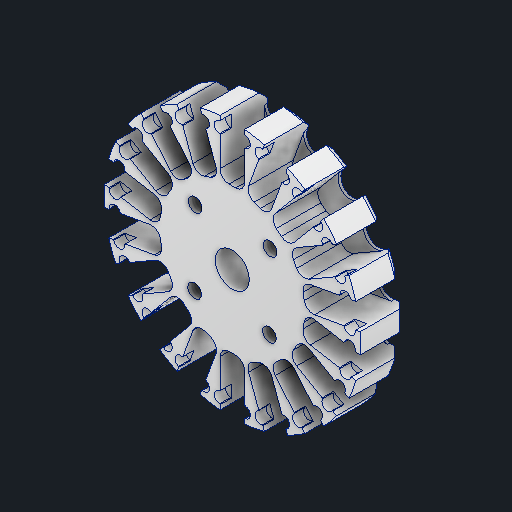
# Autodesk Inventor part: RadNeu
Saved by Autodesk Inventor 2025.2 (Build 292293000, 293)
## iProperties
Created: 2025-03-22
Part Number: RadNeu
Material: Generisch
Document SubType Name: Modeling
Designer: Faabs
Density: 1 g/cm^3
Appearance: Aluminium - flach
Author: Faabs
Autodesk Inventor part; units mm, degrees
ref_plane "YZ Plane" through (0, 0, 0) normal (1, 0, 0) x (0, 1, 0)
ref_plane "XZ Plane" through (0, 0, 0) normal (0, 1, 0) x (-1, 0, 0)
sketch "Skizze2" plane through (0, 0, 0) normal (0, -1, 0) x (1, 0, 0)
  circle A0 centre (0, 0) radius 13 construction
  circle A1 centre (0, 0) radius 23 projected
  line L0 (0, 0) -> (0, 23) construction
  line L1 (0, 23) -> (0, 13) construction
  line L2 (0, 13) -> (-0.6, 13)
  line L3 (-2.2, 14.6) -> (-2.2, 23)
  line L4 (-2.2, 23) -> (0, 23)
  line L5 (0, 23) -> (0, 13) construction
  line L6 (0, 13) -> (0.6, 13)
  line L7 (2.2, 14.6) -> (2.2, 23)
  line L8 (2.2, 23) -> (0, 23)
  arc A2 (-2.2, 14.6) -> (-0.6, 13) centre (-0.6, 14.6) ccw
  arc A3 (0.6, 13) -> (2.2, 14.6) centre (0.6, 14.6) ccw
  point P0 (2.2, 22.8945)
  point P1 (-2.2, 22.8945)
  dimension "d18" = 26
  dimension "d20" = 4.4
  dimension "d21" = 2.2
  dimension "d22" = 1.6
  dimension "d98" = 8.4
  constraints: 18 end point, 4 parallel, 4 point on circle, 4 tangent, 2 centre point, 2 perpendicular, 1 coincident, 1 collinear, 1 equal radius, 1 point on line, 1 vertical, 1 vertical alignment, 4 other
  measures "d20" distance between parallel lines of L3 L7
  measures "d21" distance between parallel lines of L0 L7
  measures "d22" radius of A2
  measures "d98" distance from line of L8 A3.centre
sketch "Skizze1" plane through (0, 0, 0) normal (0, 0, 1) x (1, 0, 0)
  line L0 (0, 0) -> (0, 8.5)
  line L1 (3.05, 0) -> (3.05, 8.5)
  line L2 (23, 0) -> (23, 8.5)
  line L3 (0, 0) -> (23, 0)
  line L4 (3.05, 8.5) -> (23, 8.5)
  dimension "d1" = 8.5
  dimension "d10" = 8.5
  dimension "d11" = 6.1
  dimension "d14" = 8.5
  dimension "d15" = 46
  constraints: 10 end point, 3 vertical, 2 horizontal
  measures "d1" distance of L0.start L0.end
  measures "d10" distance of L1.start L1.end
  measures "d11" diameter of L1 L0
  measures "d14" distance of L2.start L2.end
  measures "d15" diameter of L2 L0
revolve "Radkörper" add sketch "Skizze1" angle 360 about axis through (0, 0, 0) along (0, 1, 0)
extrude "Querrolle" cut sketch "Skizze2" against normal blind 8 contours L7 A3 L6 L2 A2 L3 A1 picked at (0, 17.4)
sketch "Skizze4" plane through (0, 0, 0) normal (0, -1, 0) x (1, 0, 0)
  line L0 (0.6, 13) -> (-0.6, 13) projected
  line L1 (0, 13) -> (0, 21) construction
  line L2 (-2.25, 22) -> (2.25, 22)
  line L3 (3.25, 21) -> (3.25, 21)
  line L4 (2.25, 20) -> (-2.25, 20)
  line L5 (-3.25, 21) -> (-3.25, 21)
  line L6 (-3.25, 22) -> (3.25, 20) construction
  line L7 (3.25, 22) -> (-3.25, 20) construction
  arc A0 (3.25, 21) -> (2.25, 22) centre (2.25, 21) ccw
  arc A1 (2.25, 20) -> (3.25, 21) centre (2.25, 21) ccw
  arc A2 (-3.25, 21) -> (-2.25, 20) centre (-2.25, 21) ccw
  arc A3 (-2.25, 22) -> (-3.25, 21) centre (-2.25, 21) ccw
  point P0 (0, 0)
  dimension "d25" = 8
  dimension "d26" = 6.5
  dimension "d27" = 2
  dimension "d28" = 1
  constraints: 14 end point, 8 point on circle, 8 point on line, 8 tangent, 4 centre point, 3 equal radius, 3 midpoint, 2 parallel, 1 horizontal, 1 perpendicular, 1 vertical
  measures "d25" distance of L1.start L1.end
  measures "d26" distance of L6.end L7.end
  measures "d27" distance of L7.start L6.end
  measures "d28" radius of A0
extrude "Achse" cut sketch "Skizze4" against normal blind 2
fillet "Rundung1" radius 0.1 4 edges at (-2.2, 1, 22) (2.2, 1, 22) (-2.2, 1, 20) (2.2, 1, 20)
pattern_circular "Runde Anordnung1" count 18 over 360 about axis through (0, -10, 0) along (0, 1, 0) of "Querrolle", "Achse", "Rundung1"
chamfer "Fasen1" distance 1.5 angle 45 1 edges at (-23, 8.5, 0)
sketch "Skizze6" plane through (0.6, 0, 14.6) normal (0, -1, 0) x (0.7071068, 0, -0.7071068)
  circle A0 centre (9.8995, -10.748) radius 9.5 construction
  line L0 (9.8995, -10.748) -> (0.7778, -1.4849) construction
  line L1 (0.4243, -1.8385) -> (1.1314, -1.1314) projected
  line L2 (9.8995, -10.748) -> (0.3998, -10.6749) construction
  point P0 (9.8264, -20.2477)
  point P1 (19.3992, -10.8211)
  point P2 (9.9726, -1.2483)
  dimension "d60" = 19
  dimension "d65" = 45
  dimension "d68" = 360
  constraints: 4 end point, 2 coincident, 1 midpoint, 8 other
  measures "d65" angle of L0 L2
hole "Bohrung1" at (-6.6656, 0, 6.769) at (6.769, 0, 6.6656) at (6.6656, 0, -6.769) at (-6.769, 0, -6.6656) direction (0, 1, 0) diameter 2.459 depth 6 tip angle 118 thread size "M3x0.5" class "6H" standard "ISO Metric profile"
sketch "Skizze12" plane through (0, 8, 0) normal (0, -1, 0) x (1, 0, 0)
  circle A0 centre (0, 0) radius 23
  line L0 (0, 23) -> (0, 20.5)
  arc A1 (-2.2, 20.5) -> (2.2, 20.5) centre (0, 20.5) ccw
  line L1 (-2.2, 14.6) -> (-2.2, 21.8897) projected
  line L2 (-2.2, 20.5) -> (-2.2, 22.8945)
  line L3 (2.2, 20.5) -> (2.2, 22.8945)
  arc A2 (-2.2955, 21.999) -> (-2.2955, 20.001) centre (-2.25, 21) ccw projected
  dimension "d85" = 46
  dimension "d86" = 2.5
  dimension "d100" = 2.2
  constraints: 6 end point, 5 point on circle, 2 centre point, 2 coincident, 2 point on line, 2 tangent, 1 parallel, 1 vertical
  measures "d85" diameter of A0
  measures "d86" distance of L0.start L0.end
  measures "d100" radius of A1
extrude "Durchbruch" cut sketch "Skizze12" against normal up to surface (0.5 mm away) contours L3 A1 L1 L2 A0 picked at (0, 21.3333)
pattern_circular "Runde Anordnung4" count 18 over 360 about axis through (0, -10, 0) along (0, 1, 0) of "Durchbruch", "Querrolle"
sketch "Skizze7" plane through (0.6, 0, 14.6) normal (0, -1, 0) x (0.7071068, 0, -0.7071068)
  circle A0 centre (0.3998, -10.6749) radius 1.2295 projected
  circle A1 centre (9.9726, -1.2483) radius 1.2295 projected
  circle A2 centre (19.3992, -10.8211) radius 1.2295 projected
  circle A3 centre (9.8264, -20.2477) radius 1.2295 projected
  point P0 (9.8995, -10.748)
  constraints: 4 coincident
hole "Durchgangsbohrung" [suppressed]
sketch "Skizze8" plane through (2.2, 8.5, -14.6) normal (0, 1, 0) x (1, 0, 0)
  line L0 (-2.2, -14.6) -> (-2.2, -17.65) construction
  circle A0 centre (-2.2, -14.6) radius 3.05 construction
  line L1 (-2.2, -14.6) -> (-4.3567, -16.7567) construction
  circle A1 centre (4.569, -21.2656) radius 1.55 projected
  line L2 (2.3236, -23.511) -> (1.5018, -20.4438)
  line L3 (1.5018, -20.4438) -> (3.7471, -18.1984)
  line L4 (3.7471, -18.1984) -> (6.8144, -19.0203)
  line L5 (6.8144, -19.0203) -> (7.6362, -22.0875)
  line L6 (7.6362, -22.0875) -> (5.3908, -24.3329)
  line L7 (5.3908, -24.3329) -> (2.3236, -23.511)
  line L8 (6.711, -10.0764) -> (3.6438, -10.8982)
  line L9 (3.6438, -10.8982) -> (1.3984, -8.6529)
  line L10 (1.3984, -8.6529) -> (2.2203, -5.5856)
  line L11 (2.2203, -5.5856) -> (5.2875, -4.7638)
  line L12 (5.2875, -4.7638) -> (7.5329, -7.0092)
  line L13 (7.5329, -7.0092) -> (6.711, -10.0764)
  line L14 (-6.7236, -5.689) -> (-5.9018, -8.7562)
  line L15 (-5.9018, -8.7562) -> (-8.1471, -11.0016)
  line L16 (-8.1471, -11.0016) -> (-11.2144, -10.1797)
  line L17 (-11.2144, -10.1797) -> (-12.0362, -7.1125)
  line L18 (-12.0362, -7.1125) -> (-9.7908, -4.8671)
  line L19 (-9.7908, -4.8671) -> (-6.7236, -5.689)
  line L20 (-11.111, -19.1236) -> (-8.0438, -18.3018)
  line L21 (-8.0438, -18.3018) -> (-5.7984, -20.5471)
  line L22 (-5.7984, -20.5471) -> (-6.6203, -23.6144)
  line L23 (-6.6203, -23.6144) -> (-9.6875, -24.4362)
  line L24 (-9.6875, -24.4362) -> (-11.9329, -22.1908)
  line L25 (-11.9329, -22.1908) -> (-11.111, -19.1236)
  point P0 (4.4656, -7.831)
  point P1 (-8.969, -7.9344)
  point P2 (-8.8656, -21.369)
  dimension "d77" = 45
  dimension "d78" = 5.5
  dimension "d81" = 360
  constraints: 52 end point, 2 point on circle, 1 coincident, 1 parallel, 1 vertical, 66 other
  measures "d77" angle of L0 L1
  measures "d78" distance between parallel lines of L6 L3
extrude "Muttern" [suppressed]
fillet "Rundung4" [suppressed]
fillet "Rundung5" [suppressed]
sketch "Skizze13" plane through (2.2, 0, 14.6) normal (0, -1, 0) x (1, 0, 0)
  circle A0 centre (-2.2, -14.6) radius 4.05
  arc A1 (-3.0292, -13.35) -> (-1.3708, -13.35) centre (-2.2, -14.6) ccw
  line L0 (-3.0292, -13.35) -> (-1.3708, -13.35)
  line L1 (-1.3268, -13.2) -> (-3.0732, -13.2)
  arc A2 (-3.0732, -13.2) -> (-1.3268, -13.2) centre (-2.2, -14.6) ccw
  dimension "d101" = 3
  dimension "d105" = 2.75
  dimension "d117" = 0.15
  constraints: 4 end point, 4 point on circle, 3 centre point, 2 coincident, 1 horizontal, 1 other
  measures "d101" diameter of A1
  measures "d117" distance between parallel lines of L0 L1
extrude "Extrusion5" [suppressed]
ref_plane "Arbeitsebene1" through (0, 0, 3) normal (0, 0, 1) x (1, 0, 0)
sketch "Skizze14" plane through (0, 0, 3) normal (0, 0, 1) x (1, 0, 0)
  line L0 (-2.2, 8.5) -> (2.2, 8.5) projected
  line L1 (0, 8.5) -> (0, 0)
  line L2 (2.5, 7.0566) -> (2.5, 4.1699)
  line L3 (2.5, 4.1699) -> (0, 2.7265)
  line L4 (0, 2.7265) -> (-2.5, 4.1699)
  line L5 (-2.5, 4.1699) -> (-2.5, 7.0566)
  line L6 (-2.5, 7.0566) -> (0, 8.5)
  line L7 (0, 8.5) -> (2.5, 7.0566)
  line L8 (2.5, 4.1699) -> (2.5, 8.5)
  line L9 (2.5, 8.5) -> (-2.5, 8.5)
  line L10 (-2.5, 8.5) -> (-2.5, 4.1699)
  circle A0 centre (0, 5.6132) radius 1.5
  dimension "d107" = 90
  dimension "d108" = 5
  dimension "d109" = 0
  dimension "d112" = 3
  constraints: 20 end point, 2 coincident, 2 point on line, 1 centre point, 1 midpoint, 1 parallel, 1 vertical, 13 other
  measures "d107" angle of L0 L2
  measures "d108" distance between parallel lines of L5 L2
  measures "d109" distance from line of L6.end L0
  measures "d112" diameter of A0
extrude "Extrusion6" [suppressed]
extrude "Extrusion7" [suppressed]
fillet "Rundung6" [suppressed]
sketch "Skizze15" plane through (0, 8.5, 0) normal (0, 1, 0) x (1, 0, 0)
  line L0 (2.155, 4.155) -> (-2.155, 4.155)
  line L1 (-4.155, 2.155) -> (-4.155, -2.155)
  line L2 (-2.155, -4.155) -> (2.155, -4.155)
  line L3 (4.155, -2.155) -> (4.155, 2.155)
  line L4 (4.155, 4.155) -> (-4.155, -4.155) construction
  line L5 (-4.155, 4.155) -> (4.155, -4.155) construction
  line L6 (4.65, 4.65) -> (-4.65, 4.65)
  line L7 (-4.65, 4.65) -> (-4.65, -4.65)
  line L8 (-4.65, -4.65) -> (4.65, -4.65)
  line L9 (4.65, -4.65) -> (4.65, 4.65)
  line L10 (4.65, 4.65) -> (-4.65, -4.65) construction
  line L11 (-4.65, 4.65) -> (4.65, -4.65) construction
  arc A0 (-2.155, 4.155) -> (-4.155, 2.155) centre (-2.155, 2.155) ccw
  arc A1 (4.155, 2.155) -> (2.155, 4.155) centre (2.155, 2.155) ccw
  arc A2 (2.155, -4.155) -> (4.155, -2.155) centre (2.155, -2.155) ccw
  arc A3 (-4.155, -2.155) -> (-2.155, -4.155) centre (-2.155, -2.155) ccw
  point P0 (0, 0)
  dimension "d122" = 9.3
  dimension "d125" = 8.31
  dimension "d130" = 2
  dimension "d131" = 8.31
  constraints: 24 end point, 9 point on line, 8 point on circle, 8 tangent, 4 centre point, 4 midpoint, 4 parallel, 3 equal radius, 2 horizontal, 2 perpendicular
  measures "d122" distance of L8.end L7.end
  measures "d125" distance of L5.start L4.end
  measures "d130" radius of A0
  measures "d131" distance between parallel lines of L1 L3
extrude "Extrusion8" cut sketch "Skizze15" against normal blind 2 contours A1 L3 A2 L2 A3 L1 A0 L0
equation "\"d10\" = d1"
equation "\"d14\" = d1"
